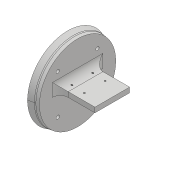
# Autodesk Inventor part: Light_Base
Saved by Autodesk Inventor 2018 (Build 220112000, 112)
## iProperties
Created: 2019-09-21
Part Number: Light_Base
Material: Generic
Document SubType Name: Modeling
Designer: Clevo
Density: 1 g/cm^3
Appearance: Default
Author: Clevo
Autodesk Inventor part; units mm, degrees
ref_plane "YZ Plane" through (0, 0, 0) normal (1, 0, 0) x (0, 1, 0)
ref_plane "XZ Plane" through (0, 0, 0) normal (0, 1, 0) x (-1, 0, 0)
sketch "Sketch1" plane through (0, 0, 0) normal (0, 1, 0) x (-1, 0, 0)
  line L0 (62.5, 0) -> (-62.5, 0)
  line L1 (-62.5, 0) -> (-17.9379, 0)
  line L2 (-17.9379, 0) -> (-17.9379, 40)
  line L3 (-62.5, 33.7372) -> (-62.5, 0)
  line L4 (-17.9379, 40) -> (10, 45) construction
  line L5 (10, 45) -> (22, 70) construction
  line L6 (22, 70) -> (62.5, 70) construction
  spline S0 degree 3 poles (-17.9379, 40) (10, 45) (22, 70) (62.5, 70) knots 1 1 1 1 2 2 2 2
  line L7 (62.5, 70) -> (62.5, 0)
  line L8 (-62.5, 33.7372) -> (-17.9379, 40)
  point P0 (0, 0)
  point P1 (0, 0)
  dimension "d0" = 125
  dimension "d1" = 40
  dimension "d2" = 45
  dimension "d3" = 45
  dimension "d4" = 10
  dimension "d5" = 70
  dimension "d6" = 22
  dimension "d7" = 70
  dimension "d9" = 98
  constraints: 12 end point, 2 horizontal, 1 coincident, 1 midpoint, 1 parallel, 1 perpendicular, 1 vertical, 1 vertical alignment, 3 other
  measures "d0" distance of L0.start L0.end
  measures "d1" distance of L1.end L2.end
  measures "d2" distance of L2.end L3.start
  measures "d3" distance from line of L0 L4.end
  measures "d4" horizontal distance of L4.end point (0, 0)
  measures "d5" vertical distance of point (0, 0) L5.end
  measures "d6" horizontal distance of point (0, 0) L5.end
  measures "d7" distance from line of L0 L6.end
  measures "d9" angle of L8 L3
revolve "Revolution1" add sketch "Sketch1" angle 360 about axis through (-62.5, 0, 0) along (1, 0, 0)
fillet "Fillet1" radius 25 1 edges at (17.9379, 0, -40)
shell "Shell1" thickness 1 removed faces 1 at (-62.5, 29.1245, -25.1102)
fillet "Fillet3" radius 0.25 2 edges at (-62.5, 0, -70) (-62.5, -0.0005, -69)
ref_plane "Work Plane1" through (0, 0, 50) normal (0, 0, 1) x (1, 0, 0)
sketch "Sketch2" plane through (0, 0, 50) normal (0, 0, 1) x (1, 0, 0)
  circle A0 centre (38, 0) radius 7.5
  point P0 (0, 0)
  dimension "d15" = 15
  dimension "d16" = 38
  constraints: 1 centre point, 1 horizontal alignment
  measures "d15" diameter of A0
  measures "d16" distance of A0.centre point (0, 0)
extrude "Extrusion1" add sketch "Sketch2" against normal up to surface round surface about axis through (40.219, 0, 0) along (-1, 0, 0) radius 36.8686 half angle 8 far side no
sketch "Sketch4" plane through (38, 0, 50) normal (0, 0, 1) x (1, 0, 0)
  line L0 (0, 4) -> (0, -4)
  circle A0 centre (0, 0) radius 7.5 projected
  point P0 (-38, 0)
  dimension "d22" = 8
  constraints: 2 end point, 1 coincident, 1 midpoint, 1 vertical
  measures "d22" distance of L0.start L0.end
hole "Hole1" at (38, 4, 50) at (38, -4, 50) direction (0, 0, -1) diameter 3.2 depth 15 tip angle 118 clearance for "Flat Head Machine Screw" size "M3" standard "Ansi Metric M Profile"
sketch "Sketch5" plane through (0, 0, 0) normal (0, 1, 0) x (-1, 0, 0)
  line L0 (-25, 4) -> (-55, 4)
  line L1 (-55, 4) -> (-55, -4)
  line L2 (-55, -4) -> (-25, -4)
  line L3 (-25, -4) -> (-25, 4)
  line L4 (-25, 4) -> (-55, -4) construction
  line L5 (-55, 4) -> (-25, -4) construction
  point P0 (0, 0)
  point P1 (-40, 0)
  point P2 (-40, 0)
  dimension "d30" = 30
  dimension "d31" = 8
  dimension "d32" = 40
  constraints: 12 end point, 3 midpoint, 2 parallel, 1 horizontal, 1 horizontal alignment, 1 perpendicular
  measures "d30" distance of L1.end L2.end
  measures "d31" distance of L0.end L1.end
  measures "d32" distance of point (0, 0) point (-40, 0)
extrude "Extrusion3" cut sketch "Sketch5" along normal through all
fillet "Fillet4" radius 2 4 edges at (55, 34.0522, -4) (55, 34.0522, 4) (25, 38.2942, -4) (25, 38.2942, 4)
pattern_circular "Circular Pattern1" count 6 over 360 about axis through (-10, 0, 0) along (1, 0, 0) of "Extrusion3", "Fillet4"
sketch "Sketch6" plane through (38, 0, 50) normal (0, 0, 1) x (1, 0, 0)
  circle A0 centre (0, 4) radius 1.6 projected
  circle A1 centre (0, -4) radius 1.6 projected
  circle A2 centre (0, 0) radius 7.5 projected
  line L0 (24.5, 33.7372) -> (24.5, -33.7372) projected
  line L1 (24.5, -4) -> (4.5, -4)
  line L2 (4.5, -4) -> (4.5, 4)
  line L3 (4.5, 4) -> (24.5, 4)
  line L4 (24.5, 4) -> (24.5, -4)
  point P0 (-38, 0)
  dimension "d39" = 20
  constraints: 8 end point, 2 horizontal alignment, 2 parallel, 1 horizontal, 1 perpendicular, 1 point on line
  measures "d39" distance of L1.start L1.end
extrude "Extrusion4" add sketch "Sketch6" against normal up to surface contours A2 L1 L2 L3 | A2 L3 L0 L1 round surface about axis through (40.219, 0, 0) along (-1, 0, 0) radius 36.8686 half angle 8 far side no picked at (5.5, 0)
fillet "Fillet5" radius 8 2 edges at (44.3443, 4, 43.0339) (44.3443, -4, 43.0339)
fillet "Fillet6" radius 8 6 edges at (55.2659, -4, 34.5229) (45.2017, -4.4374, 35.8951) (35.4005, -7.0351, 36.8808) (35.4005, 7.0351, 36.8808) (45.2017, 4.4374, 35.8951) (55.2659, 4, 34.5229)
fillet "Fillet7" radius 3 1 edges at (61.5, 0, -32.8679)
fillet "Fillet8" radius 3.5 5 edges at (62.5, 0, -33.7372) (62.5, -5.5825, 35.2293) (62.5, -4, 45.0285) (62.5, 5.5825, 35.2293) (62.5, 4, 45.0285)
ref_plane "Work Plane2" through (11.5, 0, 0) normal (-1, 0, 0) x (0, 0, 1)
sketch "Sketch7" plane through (11.5, 0, 0) normal (-1, 0, 0) x (0, 0, 1)
  spline S0 degree 8 poles (40.5203, 0) (40.5203, 3.9771) (40.0742, 7.9568) (39.1809, 11.8766) (37.8512, 15.6785) (36.1031, 19.307) (33.963, 22.7104) (31.4644, 25.8399) (25.8175, 31.4869) (22.6603, 34.003) (19.2253, 36.1545) (15.5622, 37.907) (11.7245, 39.2338) (7.7686, 40.1166) (3.7542, 40.5447) (-4.1998, 40.4947) (-8.1448, 40.0309) (-12.0286, 39.1275) (-15.7945, 37.7951) (-19.3887, 36.0517) (-22.7605, 33.923) (-25.8624, 31.4419) (-31.4644, 25.8399) (-33.963, 22.7104) (-36.1031, 19.307) (-37.8512, 15.6785) (-39.1809, 11.8766) (-40.0742, 7.9568) (-40.5203, 3.9771) (-40.5203, -3.9771) (-40.0742, -7.9568) (-39.1809, -11.8766) (-37.8512, -15.6785) (-36.1031, -19.307) (-33.963, -22.7104) (-31.4644, -25.8399) (-25.8399, -31.4644) (-22.7104, -33.963) (-19.307, -36.1031) (-15.6785, -37.8512) (-11.8766, -39.1809) (-7.9568, -40.0742) (-3.9771, -40.5203) (3.9771, -40.5203) (7.9568, -40.0742) (11.8766, -39.1809) (15.6785, -37.8512) (19.307, -36.1031) (22.7104, -33.963) (25.8399, -31.4644) (31.4644, -25.8399) (33.963, -22.7104) (36.1031, -19.307) (37.8512, -15.6785) (39.1809, -11.8766) (40.0742, -7.9568) (40.5203, -3.9771) (40.5203, 0) knots 0 0 0 0 0 0 0 0 0 0.125 0.125 0.125 0.125 0.125 0.125 0.125 0.250999 0.250999 0.250999 0.250999 0.250999 0.250999 0.250999 0.375 0.375 0.375 0.375 0.375 0.375 0.375 0.5 0.5 0.5 0.5 0.5 0.5 0.5 0.625 0.625 0.625 0.625 0.625 0.625 0.625 0.75 0.75 0.75 0.75 0.75 0.75 0.75 0.875 0.875 0.875 0.875 0.875 0.875 0.875 1 1 1 1 1 1 1 1 1 projected
  point P0 (0, 0)
  constraints: 2 other
extrude "Extrusion5" add sketch "Sketch7" against normal blind 10 separate body
sketch "Sketch10" plane through (0, 0, 0) normal (0, 0, 1) x (1, 0, 0)
  line L0 (-92.8724, 88.0568) -> (92.8724, 88.0568)
  line L1 (92.8724, 88.0568) -> (92.8724, -88.0568)
  line L2 (92.8724, -88.0568) -> (-92.8724, -88.0568)
  line L3 (-92.8724, -88.0568) -> (-92.8724, 88.0568)
  line L4 (-92.8724, 88.0568) -> (92.8724, -88.0568) construction
  line L5 (92.8724, 88.0568) -> (-92.8724, -88.0568) construction
  point P0 (0, 0)
  constraints: 12 end point, 2 midpoint, 2 parallel, 1 horizontal, 1 perpendicular
extrude "Extrusion6" cut sketch "Sketch10" along normal through all bodies 1
sketch "Sketch11" plane through (0, 0, 0) normal (0, 0, 1) x (1, 0, 0)
  spline S0 degree 7 poles (-62.5, -69.2497) (-62.5, -69.2245) (-62.497, -69.198) (-62.4906, -69.1709) (-62.4802, -69.1438) (-62.4658, -69.1178) (-62.4479, -69.094) (-62.4061, -69.0522) (-62.3824, -69.0342) (-62.3565, -69.0197) (-62.3294, -69.0093) (-62.3023, -69.0028) (-62.2759, -68.9997) (-62.2506, -68.9997) knots 0 0 0 0 0 0 0 0 0.5 0.5 0.5 0.5 0.5 0.5 1 1 1 1 1 1 1 1 projected
  line L0 (-62.5, -69.7497) -> (-62.5, -69.2497) projected
  line L1 (25, -39.0075) -> (18.4739, -39.9247) projected
  line L2 (25, -37.9977) -> (25, -39.0075) projected
  line L3 (18.3347, -38.9344) -> (25, -37.9977) projected
  spline S1 degree 2 poles (17.0201, -39.1537) (17.6746, -39.0272) (18.3347, -38.9344) knots 0 0 0 1 1 1 weights 1 0.999671 1 projected
  spline S2 degree 5 poles (-62.2506, -68.9997) (-58.903, -68.9911) (-55.5555, -68.8386) (-52.217, -68.5235) (-48.9002, -68.0326) (-42.8529, -66.789) (-40.1108, -66.0896) (-37.4058, -65.2564) (-34.7449, -64.2947) (-28.9803, -61.9196) (-25.8977, -60.4535) (-22.8877, -58.8467) (-19.9377, -57.1382) (-14.6946, -53.9784) (-12.3908, -52.5452) (-10.0917, -51.104) (-7.7809, -49.6817) (-1.2389, -45.8402) (3.0621, -43.524) (7.5426, -41.5382) (12.2328, -40.0788) (17.0201, -39.1537) knots 0 0 0 0 0 0 0.194984 0.194984 0.194984 0.194984 0.359594 0.359594 0.359594 0.359594 0.558121 0.558121 0.558121 0.558121 0.716155 0.716155 0.716155 0.716155 1 1 1 1 1 1 projected
  line L4 (25, -37.9977) -> (25, -56.9984)
  line L5 (25, -56.9984) -> (-40.1862, -72.9396)
  line L6 (-40.1862, -72.9396) -> (-62.5, -74.7707)
  line L7 (-62.5, -74.7707) -> (-62.5, -69.7497)
  line L8 (-88.168, 0) -> (87.6113, 0) projected
  point P0 (0, 0)
  constraints: 8 end point, 1 parallel, 1 vertical, 6 other
revolve "Revolution2" cut sketch "Sketch11" angle 360 about axis through (-10, 0, 0) along (1, 0, 0) bodies 2
sketch "Sketch12" plane through (0, 0, 0) normal (0, 0, 1) x (1, 0, 0)
  line L0 (-70.0381, 73.5) -> (70.0381, 73.5)
  line L1 (70.0381, 73.5) -> (70.0381, -73.5)
  line L2 (70.0381, -73.5) -> (-70.0381, -73.5)
  line L3 (-70.0381, -73.5) -> (-70.0381, 73.5)
  line L4 (-70.0381, 73.5) -> (70.0381, -73.5) construction
  line L5 (70.0381, 73.5) -> (-70.0381, -73.5) construction
  point P0 (0, 0)
  constraints: 12 end point, 2 midpoint, 2 parallel, 1 horizontal, 1 perpendicular
extrude "Extrusion7" cut sketch "Sketch12" against normal through all bodies 1
sketch "Sketch13" plane through (11.5, 0, 0) normal (-1, 0, 0) x (0, 0, 1)
  line L0 (-20, -20) -> (20, -20)
  line L1 (20, -20) -> (20, 20)
  line L2 (20, 20) -> (-20, 20)
  line L3 (-20, 20) -> (-20, -20)
  line L4 (-20, -20) -> (20, 20) construction
  line L5 (20, -20) -> (-20, 20) construction
  point P0 (0, 0)
  dimension "d54" = 40
  dimension "d55" = 40
  constraints: 12 end point, 2 midpoint, 2 parallel, 1 horizontal, 1 perpendicular
  measures "d54" distance of L0.end L1.end
  measures "d55" distance of L0.start L0.end
hole "Hole2" at (11.5, 20, 20) at (11.5, 20, -20) at (11.5, -20, -20) at (11.5, -20, 20) direction (1, 0, 0) diameter 3.4 end through all bodies 2 clearance for "Flat Head Machine Screw" size "M3" standard "Ansi Metric M Profile"
sketch "Sketch14" plane through (11.5, 0, 0) normal (-1, 0, 0) x (0, 0, 1)
  line L0 (0, 12.5) -> (-5, 12.5)
  line L1 (-5, 12.5) -> (-5, -12.5)
  line L2 (-5, -12.5) -> (0, -12.5)
  line L3 (0, -12.5) -> (0, 12.5)
  point P0 (0, 0)
  point P1 (0, 0)
  dimension "d63" = 5
  dimension "d64" = 25
  constraints: 8 end point, 2 parallel, 1 coincident, 1 horizontal, 1 midpoint, 1 perpendicular
  measures "d63" distance of L1.end L2.end
  measures "d64" distance of L0.end L1.end
extrude "Extrusion8" cut sketch "Sketch14" against normal through all bodies 2
fillet "Fillet9" radius 2 4 edges at (16.5, 12.5, 0) (16.5, -12.5, 0) (16.5, -12.5, -5) (16.5, 12.5, -5)
sketch "Sketch15" plane through (21.5, 0, 0) normal (1, 0, 0) x (0, 0, -1)
  line L0 (5, 10.5) -> (5, -10.5) projected
  arc A0 (3, -12.5) -> (5, -10.5) centre (3, -10.5) ccw projected
  line L1 (3, -12.5) -> (2, -12.5) projected
  arc A1 (0, -10.5) -> (2, -12.5) centre (2, -10.5) ccw projected
  line L2 (0, -10.5) -> (0, 10.5) projected
  arc A2 (2, 12.5) -> (0, 10.5) centre (2, 10.5) ccw projected
  line L3 (2, 12.5) -> (3, 12.5) projected
  arc A3 (5, 10.5) -> (3, 12.5) centre (3, 10.5) ccw projected
  circle A4 centre (20, -20) radius 1.7 projected
  circle A5 centre (-20, 20) radius 1.7 projected
  circle A6 centre (20, 20) radius 1.7 projected
  circle A7 centre (-20, -20) radius 1.7 projected
  circle A8 centre (0, 0) radius 38.4896 projected
  line L4 (-5, -17.5) -> (0, -17.5)
  line L5 (0, -17.5) -> (0, 17.5)
  line L6 (0, 17.5) -> (-5, 17.5)
  line L7 (-5, 17.5) -> (-5, -17.5)
  point P0 (0, 0)
  point P1 (0, 0)
  dimension "d68" = 5
  dimension "d69" = 35
  constraints: 8 end point, 2 midpoint, 2 parallel, 1 horizontal, 1 perpendicular
  measures "d68" distance of L5.end L6.end
  measures "d69" distance of L6.end L4.start
extrude "Extrusion9" add sketch "Sketch15" along normal blind 35 contours L2 L5 L4 L7 L6 bodies 2
fillet "Fillet10" radius 8 3 edges at (21.5, 0, 5) (21.5, -17.5, 2.5) (21.5, 17.5, 2.5)
sketch "Sketch16" plane through (11.5, -10.5, 0) normal (0, 0, -1) x (-1, 0, 0)
  line L0 (-45, -7) -> (-45, 28) projected
  line L1 (-27.25, 0) -> (-14.75, 0)
  line L2 (-14.75, 0) -> (-14.75, 21)
  line L3 (-14.75, 21) -> (-27.25, 21)
  line L4 (-27.25, 21) -> (-27.25, 0)
  line L5 (-27.25, 0) -> (-14.75, 21) construction
  line L6 (-14.75, 0) -> (-27.25, 21) construction
  point P0 (11.5, 10.5)
  point P1 (-21, 10.5)
  point P2 (-45, 10.5)
  point P3 (-21, 10.5)
  dimension "d73" = 12.5
  dimension "d74" = 21
  dimension "d75" = 24
  constraints: 12 end point, 4 midpoint, 2 parallel, 1 horizontal, 1 horizontal alignment, 1 perpendicular
  measures "d73" distance of L2.end L3.end
  measures "d74" distance of L3.end L1.start
  measures "d75" distance from line of L0 point (-21, 10.5)
hole "Hole3" at (38.75, -10.5, 0) at (38.75, 10.5, 0) at (26.25, 10.5, 0) at (26.25, -10.5, 0) direction (0, 0, 1) diameter 1.567 end through all bodies 2 thread size "M2x0.4" class "6H" standard "ANSI Metric M Profile"
equation "\"d55\" = d54"
body "Solid1"
body "Solid3"
